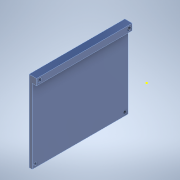
# Autodesk Inventor part: Part2
Saved by Autodesk Inventor 2022 (Build 260153000, 153)
## iProperties
Created: 2022-04-28
Part Number: Part2
Material: Generic
Document SubType Name: Modeling
Designer: Oana
Density: 1 g/cm^3
Appearance: Flaked Satin - Blue
Author: Oana
Autodesk Inventor part; units mm, degrees
ref_plane "YZ Plane" through (0, 0, 0) normal (1, 0, 0) x (0, 1, 0)
ref_plane "XZ Plane" through (0, 0, 0) normal (0, 1, 0) x (-1, 0, 0)
ref_plane "XY Plane" through (0, 0, 0) normal (0, 0, 1) x (1, 0, 0)
sketch "Sketch1" plane through (0, 0, 0) normal (1, 0, 0) x (0, 1, 0)
  line L0 (59.5474, 107.5539) -> (-16.4526, 107.5539)
  line L1 (-16.4526, 107.5539) -> (-16.4526, 17.5539)
  line L2 (-16.4526, 17.5539) -> (59.5474, 17.5539)
  line L3 (59.5474, 17.5539) -> (59.5474, 107.5539)
  point P0 (0, 0)
  dimension "d0" = 90
  dimension "d1" = 76
  constraints: 8 end point, 2 parallel, 1 horizontal, 1 perpendicular
  measures "d0" distance of L2.end L0.start
  measures "d1" distance of L1.end L2.end
extrude "Extrusion1" add sketch "Sketch1" along normal blind 3
sketch "Sketch2" plane through (3, 0, 0) normal (1, 0, 0) x (0, 0, -1)
  point P0 (0, 0)
sketch "Sketch3" plane through (3, 0, 0) normal (1, 0, 0) x (0, 0, -1)
  line L0 (-107.5539, -16.4526) -> (-17.5539, -16.4526) projected
  line L1 (-17.5539, -16.4526) -> (-17.5539, 59.5474) projected
  line L2 (-17.5539, 59.5474) -> (-107.5539, 59.5474) projected
  line L3 (-107.5539, 59.5474) -> (-107.5539, -16.4526) projected
  line L4 (-107.5539, 59.5474) -> (-17.5539, 59.5474)
  line L5 (-17.5539, 59.5474) -> (-17.5539, 53.5474)
  line L6 (-17.5539, 53.5474) -> (-107.5539, 53.5474)
  line L7 (-107.5539, 53.5474) -> (-107.5539, 59.5474)
  point P0 (0, 0)
  dimension "d4" = 6
  constraints: 8 end point, 2 parallel, 1 horizontal, 1 perpendicular, 1 point on line
  measures "d4" distance between parallel lines of L2 L6
extrude "Extrusion2" add sketch "Sketch3" along normal blind 4 contours L3 L2 L1 L6
sketch "Sketch5" plane through (0, 0, 0) normal (-1, 0, 0) x (0, 0, 1)
  line L0 (107.5539, -16.4526) -> (17.5539, -16.4526) projected
  line L1 (107.5539, 59.5474) -> (107.5539, -16.4526) projected
  line L2 (17.5539, 59.5474) -> (107.5539, 59.5474) projected
  line L3 (17.5539, -16.4526) -> (17.5539, 59.5474) projected
  line L4 (17.5539, -16.4526) -> (20.5539, -16.4526)
  line L5 (20.5539, -16.4526) -> (20.5539, -13.4526) construction
  line L6 (20.5539, -13.4526) -> (17.5539, -13.4526) construction
  line L7 (17.5539, -13.4526) -> (17.5539, -16.4526)
  circle A0 centre (20.5539, -13.4526) radius 1.5
  line L8 (107.5539, -16.4526) -> (104.5539, -16.4526)
  line L9 (104.5539, -16.4526) -> (104.5539, -13.4526)
  line L10 (104.5539, -13.4526) -> (107.5539, -13.4526)
  line L11 (107.5539, -13.4526) -> (107.5539, -16.4526)
  line L12 (17.5539, 59.5474) -> (20.5539, 59.5474)
  line L13 (20.5539, 59.5474) -> (20.5539, 56.5474)
  line L14 (20.5539, 56.5474) -> (17.5539, 56.5474)
  line L15 (17.5539, 56.5474) -> (17.5539, 59.5474)
  line L16 (107.5539, 59.5474) -> (104.5539, 59.5474)
  line L17 (104.5539, 59.5474) -> (104.5539, 56.5474)
  line L18 (104.5539, 56.5474) -> (107.5539, 56.5474)
  line L19 (107.5539, 56.5474) -> (107.5539, 59.5474)
  circle A1 centre (20.5539, 56.5474) radius 1.8641
  circle A2 centre (104.5539, 56.5474) radius 1.8641
  circle A3 centre (104.5539, -13.4526) radius 1.5
  point P0 (0, 0)
  dimension "d7" = 3
  dimension "d9" = 3
  constraints: 32 end point, 8 parallel, 6 equal length, 4 centre point, 4 coincident, 4 horizontal, 4 perpendicular, 2 equal radius, 1 point on line
  measures "d7" distance of L5.end L6.end
  measures "d9" diameter of A0
extrude "Extrusion3" cut sketch "Sketch5" against normal up to surface (7 mm away) contours A3 L10 L9 | L9 L10 A3 | A2 L17 L18 | L18 L17 A2 | A1 L13 L14 | L14 L13 A1 | A0
body "Solid1"
